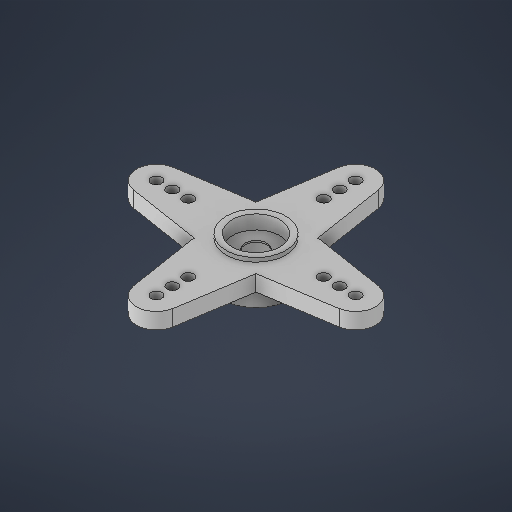
# Autodesk Inventor part: MMAE 232 CAD Assignment 2 Servo Horn 5-Nicholas Skiba
Saved by Autodesk Inventor 2026.1 (Build 301233000, 233)
## iProperties
Created: 2025-08-27
Part Number: MMAE 232 CAD Assignment 2 Servo Horn 5-Nicholas Skiba
Material: Generic
Document SubType Name: Modeling
Designer: Nick
Density: 1 g/cm^3
Appearance: Default
Author: Nick
Autodesk Inventor part; units mm, degrees
ref_plane "YZ Plane" through (0, 0, 0) normal (1, 0, 0) x (0, 1, 0)
ref_plane "XZ Plane" through (0, 0, 0) normal (0, 1, 0) x (-1, 0, 0)
ref_plane "XY Plane" through (0, 0, 0) normal (0, 0, 1) x (1, 0, 0)
sketch "Sketch1" plane through (0, 0, 0) normal (0, 1, 0) x (-1, 0, 0)
  circle A0 centre (0, 0) radius 10.5 construction
  circle A1 centre (0, 0) radius 12.5 construction
  circle A2 centre (0, 0) radius 8.5 construction
  circle A3 centre (12.5, 0) radius 2.5
  circle A4 centre (12.5, 0) radius 0.675
  circle A5 centre (10.5, 0) radius 0.675
  circle A6 centre (8.5, 0) radius 0.675
  line L0 (0, 16.4462) -> (0, -19.2601)
  circle A7 centre (0, 12.5) radius 0.675
  circle A8 centre (0, 10.5) radius 0.675
  circle A9 centre (0, 12.5) radius 2.5
  circle A10 centre (0, 8.5) radius 0.675
  circle A11 centre (-12.5, 0) radius 0.675
  circle A12 centre (-10.5, 0) radius 0.675
  circle A13 centre (-12.5, 0) radius 2.5
  circle A14 centre (-8.5, 0) radius 0.675
  circle A15 centre (0, -12.5) radius 0.675
  circle A16 centre (0, -10.5) radius 0.675
  circle A17 centre (0, -12.5) radius 2.5
  circle A18 centre (0, -8.5) radius 0.675
  line L1 (0, 0) -> (7.0711, -7.0711) construction
  line L2 (0, 0) -> (10, 0) construction
  line L3 (0, 0) -> (7.0711, 7.0711) construction
  line L4 (0, 0) -> (10, 0) construction
  line L5 (0, 0) -> (7.0711, -7.0711) construction
  line L6 (0, 0) -> (10, 0) construction
  line L7 (0, 0) -> (-7.0711, -7.0711) construction
  line L8 (0, 0) -> (10, 0) construction
  line L9 (3.8872, -3.8872) -> (12.8889, -2.4696)
  line L10 (3.8872, -3.8872) -> (2.4696, -12.8889)
  line L11 (3.8872, 3.8872) -> (2.4696, 12.8889)
  line L12 (3.8872, 3.8872) -> (12.8889, 2.4696)
  line L13 (-3.8872, 3.8872) -> (-12.8889, 2.4696)
  line L14 (-3.8872, 3.8872) -> (-2.4696, 12.8889)
  line L15 (-3.8872, -3.8872) -> (-2.4696, -12.8889)
  line L16 (-3.8872, -3.8872) -> (-12.8889, -2.4696)
  point P0 (13.5701, 2.2594)
  point P1 (14.0204, -1.9845)
  point P2 (-2.2594, 13.5701)
  point P3 (1.9845, 14.0204)
  point P4 (-13.5701, -2.2594)
  point P5 (-14.0204, 1.9845)
  point P6 (2.2594, -13.5701)
  point P7 (-1.9845, -14.0204)
  dimension "d0" = 21
  dimension "d1" = 25
  dimension "d2" = 17
  dimension "d3" = 5
  dimension "d4" = 1.35
  dimension "d5" = 1.35
  dimension "d6" = 1.35
  dimension "d9" = 360
  dimension "d11" = 10
  dimension "d12" = 45
  dimension "d13" = 10
  dimension "d14" = 45
  dimension "d15" = 10
  dimension "d16" = 45
  dimension "d17" = 10
  dimension "d18" = 135
  dimension "d19" = 107.9
  dimension "d20" = 12.5
  dimension "d21" = 10.5
  dimension "d22" = 2
  dimension "d23" = 8.5
  dimension "d24" = 8.5
  dimension "d25" = 10.5
  dimension "d26" = 12.5
  dimension "d27" = 12.5
  dimension "d30" = 360
  constraints: 34 end point, 16 centre point, 10 point on circle, 7 coincident, 4 equal length, 4 horizontal, 3 horizontal alignment, 2 tangent, 1 point on line, 1 vertical, 68 other
  measures "d3" diameter of A3
  measures "d4" diameter of A4
  measures "d5" diameter of A5
  measures "d6" diameter of A6
  measures "d11" distance of L1.start L1.end
  measures "d12" angle of L1 L2
  measures "d13" distance of L1.start L3.end
  measures "d14" angle of L4 L3
  measures "d15" distance of L1.start L1.end
  measures "d16" angle of L5 L6
  measures "d17" distance of L1.start L7.end
  measures "d18" angle of L7 L8
  measures "d19" angle of L9 L10
  measures "d20" distance of point (0, 0) A15.centre
  measures "d21" distance of point (0, 0) A16.centre
  measures "d22" distance of A18.centre A16.centre
  measures "d23" distance of point (0, 0) A18.centre
  measures "d24" horizontal distance of A6.centre A18.centre
  measures "d25" distance of point (0, 0) A5.centre
  measures "d26" distance of point (0, 0) A3.centre
  measures "d27" horizontal distance of A3.centre A15.centre
extrude "Extrusion1" add sketch "Sketch1" along normal blind 2 contours A3 A5 | A3 A5 L9 L10 A17 A16 L0 A18 A10 A8 A9 L11 L12 | A9 A8 L0 A7 | A17 L0 A15 A16 | L0 A7 A8 A9 | A17 A16 L0 A15 | A9 A8 L0 A10 A18 A16 A17 L15 L16 A13 A12 L13 L14 | A13 A12 picked at (11.2959, 0.9935) picked at (-11.3085, -0.9832)
sketch "Sketch2" plane through (0, 2, 0) normal (0, 1, 0) x (1, 0, 0)
  circle A0 centre (0, 0) radius 3.74
  circle A1 centre (0, 0) radius 2.99
  circle A2 centre (0, 0) radius 1.37
  dimension "d34" = 7.48
  dimension "d35" = 5.98
  dimension "d36" = 2.74
  constraints: 3 centre point, 3 coincident
  measures "d34" diameter of A0
  measures "d35" diameter of A1
  measures "d36" diameter of A2
extrude "Extrusion2" add sketch "Sketch2" along normal blind 0.5 contours A0
extrude "Extrusion3" cut sketch "Sketch2" against normal blind 1.25 contours A1
extrude "Extrusion4" cut sketch "Sketch2" against normal through all contours A2
sketch "Sketch3" plane through (0, 0, 0) normal (0, -1, 0) x (1, 0, 0)
  circle A0 centre (0, 0) radius 1.37 projected
  circle A1 centre (0, 0) radius 2.75
  circle A2 centre (0, 0) radius 4.45
  dimension "d43" = 5.5
  dimension "d44" = 8.9
  constraints: 2 centre point, 2 coincident
  measures "d43" diameter of A1
  measures "d44" diameter of A2
extrude "Extrusion5" add sketch "Sketch3" along normal blind 2.44 contours A2
extrude "Extrusion6" cut sketch "Sketch3" against normal blind 0.56 contours A1
body "Solid1"
